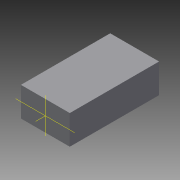
# Autodesk Inventor part: test
Saved by Autodesk Inventor 2014 (Build 180170000, 170)
## iProperties
Created: 2014-11-21
Part Number: test
Material: Generic
Document SubType Name: Modeling
Designer: KriMag
Density: 1 g/cm^3
Appearance: Default
Author: KriMag
Autodesk Inventor part; units mm, degrees
ref_plane "YZ Plane" through (0, 0, 0) normal (1, 0, 0) x (0, 1, 0)
ref_plane "XZ Plane" through (0, 0, 0) normal (0, 1, 0) x (-1, 0, 0)
ref_plane "XY Plane" through (0, 0, 0) normal (0, 0, 1) x (1, 0, 0)
sketch "Sketch2" plane through (0, 0, 0) normal (0, 1, 0) x (-1, 0, 0)
  line L0 (-5.2, -3.1) -> (5.2, -3.1)
  line L1 (5.2, -3.1) -> (5.2, 3.1)
  line L2 (5.2, 3.1) -> (-5.2, 3.1)
  line L3 (-5.2, 3.1) -> (-5.2, -3.1)
  line L4 (-5.2, -3.1) -> (5.2, 3.1) construction
  line L5 (5.2, -3.1) -> (-5.2, 3.1) construction
  point P0 (0, 0)
  dimension "d10" = 10.4
  dimension "d11" = 6.2
  constraints: 12 end point, 2 midpoint, 2 parallel, 1 horizontal, 1 perpendicular
  measures "d10" distance of L2.end L1.end
  measures "d11" distance of L1.end L0.end
extrude "Extrusion1" add sketch "Sketch2" along normal blind 14
sketch "Sketch3" plane through (0, 14, 0) normal (0, 1, 0) x (1, 0, 0)
  line L0 (5.2, 3.1) -> (-5.2, 3.1) projected
  line L1 (-5.2, 3.1) -> (-5.2, -3.1) projected
  line L2 (-4.2, 2.1) -> (4, 2.1)
  line L3 (4, 2.1) -> (4, 0.5)
  line L4 (4, 0.5) -> (-4.2, 0.5)
  line L5 (-4.2, 0.5) -> (-4.2, 2.1)
  point P0 (0, 0)
  dimension "d14" = 8.2
  dimension "d15" = 1.6
  dimension "d16" = 1
  dimension "d17" = 1
  constraints: 8 end point, 2 parallel, 1 horizontal, 1 perpendicular
  measures "d14" distance of L3.end L4.end
  measures "d15" distance of L2.end L3.end
  measures "d16" distance between parallel lines of L0 L2
  measures "d17" distance between parallel lines of L1 L5
extrude "Extrusion2" cut sketch "Sketch3" against normal blind 0.5
sketch "Sketch4" plane through (0, 14, 0) normal (0, 1, 0) x (1, 0, 0)
  line L0 (-4.2, 2.1) -> (4, 2.1) projected
  line L1 (-5.2, -3.1) -> (5.2, -3.1) projected
  line L2 (-4.2, 0.5) -> (4, 0.5)
  line L3 (4, 0.5) -> (4, -2.1)
  line L4 (4, -2.1) -> (-4.2, -2.1)
  line L5 (-4.2, -2.1) -> (-4.2, 0.5)
  point P0 (0, 0)
  dimension "d20" = 1
  constraints: 8 end point, 3 parallel, 1 horizontal, 1 perpendicular
  measures "d20" distance between parallel lines of L4 L1
extrude "Extrusion3" cut sketch "Sketch4" against normal blind 12
sketch "Sketch5" plane through (0, 14, 0) normal (0, 1, 0) x (1, 0, 0)
  line L0 (-5.2, 3.1) -> (5.2, 3.1)
  line L1 (5.2, 3.1) -> (5.2, -3.1)
  line L2 (5.2, -3.1) -> (-5.2, -3.1)
  line L3 (-5.2, -3.1) -> (-5.2, 3.1)
  line L4 (4, -2.1) -> (-4.2, -2.1)
  line L5 (-4.2, -2.1) -> (-4.2, 2.1)
  line L6 (-4.2, 2.1) -> (4, 2.1)
  line L7 (4, 2.1) -> (4, -2.1)
  point P0 (0, 0)
  constraints: 16 end point, 4 parallel, 2 horizontal, 2 perpendicular
extrude "Extrusion4" add sketch "Sketch5" along normal blind 5
body "Solid1"
